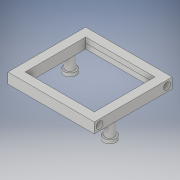
# Autodesk Inventor part: yaxis_platform
Saved by Autodesk Inventor 2019 (Build 230136000, 136)
## iProperties
Created: 2020-02-02
Material: Generic
Document SubType Name: Modeling
Designer: Nishant
Density: 1 g/cm^3
Appearance: Default
Author: Nishant
Autodesk Inventor part; units mm, degrees
ref_plane "YZ Plane" through (0, 0, 0) normal (1, 0, 0) x (0, 1, 0)
ref_plane "XZ Plane" through (0, 0, 0) normal (0, 1, 0) x (-1, 0, 0)
ref_plane "XY Plane" through (0, 0, 0) normal (0, 0, 1) x (1, 0, 0)
sketch "Sketch1" plane through (0, 0, 0) normal (0, 1, 0) x (-1, 0, 0)
  line L0 (25, 0) -> (25, 45)
  line L1 (25, 45) -> (-25, 45)
  line L2 (-25, 45) -> (-25, 0)
  line L3 (25, 0) -> (-25, 0)
  line L4 (20, 5) -> (-20, 5)
  line L5 (-20, 5) -> (-20, 40)
  line L6 (-20, 40) -> (20, 40)
  line L7 (20, 40) -> (20, 5)
  point P0 (0, 0)
  dimension "d2" = 45
  dimension "d3" = 50
  dimension "d4" = 45
  dimension "d5" = 50
  dimension "d9" = 35
  dimension "d10" = 40
  dimension "d11" = 35
  constraints: 16 end point, 3 perpendicular, 2 horizontal, 1 vertical
  measures "d2" distance of L0.start L0.end
  measures "d3" distance of L0.end L1.end
  measures "d4" distance of L1.end L2.end
  measures "d5" distance of L0.start L2.end
  measures "d9" distance of L4.end L5.end
  measures "d10" distance of L5.end L6.end
  measures "d11" distance of L6.end L4.start
extrude "Extrusion1" add sketch "Sketch1" along normal blind 6
sketch "Sketch2" plane through (0, 0, 0) normal (0, -1, 0) x (1, 0, 0)
  line L0 (25, 45) -> (25, 0) projected
  line L1 (-25, 45) -> (25, 45) projected
  circle A0 centre (22.5, 33.5) radius 2.5
  line L2 (-25, 0) -> (-25, 45) projected
  line L3 (25, 0) -> (-25, 0) projected
  circle A1 centre (-22.5, 11.5) radius 2.5
  point P0 (0, 0)
  dimension "d16" = 5
  dimension "d19" = 5
  constraints: 2 centre point
  measures "d16" diameter of A0
  measures "d19" diameter of A1
extrude "Extrusion2" add sketch "Sketch2" along normal blind 7.5 contours A1 | A0
sketch "Sketch3" plane through (22.5, -7.5, 33.5) normal (0, -1, 0) x (1, 0, 0)
  circle A0 centre (0, 0) radius 3.5
  point P0 (-22.5, -33.5)
  dimension "d22" = 7
  constraints: 1 centre point
  measures "d22" diameter of A0
sketch "Sketch4" plane through (-22.5, -7.5, 11.5) normal (0, -1, 0) x (1, 0, 0)
  circle A0 centre (0, 0) radius 3.5
  point P0 (22.5, -11.5)
  dimension "d23" = 7
  constraints: 1 centre point
  measures "d23" diameter of A0
extrude "Extrusion3" add sketch "Sketch4" along normal blind 2
extrude "Extrusion4" add sketch "Sketch3" along normal blind 2
sketch "Sketch6" plane through (25, 0, 0) normal (1, 0, 0) x (0, 0, -1)
  line L0 (0, 0) -> (0, 6)
  line L1 (0, 0) -> (0, 6) projected
  line L2 (-45, 0) -> (-45, 6)
  circle A0 centre (-42, 3) radius 2
  circle A1 centre (-3, 3) radius 2
  dimension "d41" = 6
  dimension "d44" = 4
  dimension "d45" = 4
  constraints: 4 end point, 2 centre point
  measures "d41" distance of L0.start L0.end
  measures "d44" diameter of A0
  measures "d45" diameter of A1
hole "Hole2" at (25, 3, 42) at (25, 3, 3) direction (-1, 0, 0) diameter 4 end through all both
body "Solid1"
